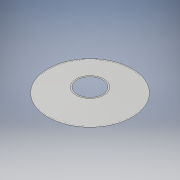
# Autodesk Inventor part: PropellorGuardTop
Saved by Autodesk Inventor 2019 (Build 230136000, 136)
## iProperties
Created: 2020-01-19
Part Number: PropellorGuardTop
Material: Generic
Document SubType Name: Modeling
Designer: 18186
Density: 1 g/cm^3
Appearance: Default
Author: 18186
Autodesk Inventor part; units mm, degrees
ref_plane "YZ Plane" through (0, 0, 0) normal (1, 0, 0) x (0, 1, 0)
ref_plane "XZ Plane" through (0, 0, 0) normal (0, 1, 0) x (-1, 0, 0)
ref_plane "Work Plane1" through (0, 0, 50.8) normal (0, 0, 1) x (1, 0, 0)
sketch "Sketch5" plane through (0, 0, 0) normal (0, 0, 1) x (1, 0, 0)
  line L0 (0, 0) -> (-419.1, 0)
  line L1 (0, 0) -> (0, 50.8)
  line L2 (0, 50.8) -> (-139.7, 50.8)
  line L3 (-139.7, 50.8) -> (-419.1, 0)
  dimension "d26" = 419.1
  dimension "d27" = 50.8
  dimension "d28" = 139.7
  constraints: 8 end point, 2 horizontal, 1 vertical
  measures "d26" distance of L0.start L0.end
  measures "d27" distance of L0.start L1.end
  measures "d28" distance of L1.end L2.end
revolve "Revolution1" add sketch "Sketch5" angle 360 about axis through (0, 0, 0) along (0, 1, 0)
sketch "Sketch6" plane through (0, 0, 0) normal (0, -1, 0) x (1, 0, 0)
  circle A0 centre (0, 0) radius 406.4
  dimension "d30" = 812.8
  constraints: 1 centre point, 1 coincident
  measures "d30" diameter of A0
sketch "Sketch7" plane through (0, 50.8, 0) normal (0, 1, 0) x (1, 0, 0)
  circle A0 centre (0, 0) radius 127
  dimension "d31" = 254
  constraints: 1 centre point, 1 coincident
  measures "d31" diameter of A0
loft "Loft1" cut profiles "Sketch6", "Sketch7"
body "Solid3"
